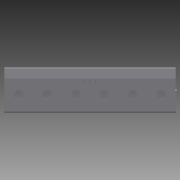
# Autodesk Inventor part: obodowka
Saved by Autodesk Inventor 2015 (Build 190159000, 159)
## iProperties
Created: 2015-09-19
Part Number: obodowka
Material: Generic
Document SubType Name: Sheet Metal
Designer: Komp
Density: 1 g/cm^3
Sheet Metal Rule: Default_mm
Appearance: Default
Flat Pattern Width: 17.082 cm
Flat Pattern Length: 30 cm
Flat Pattern Area: 512.46 cm^2
Sheet Metal Width: 170,820 mm
Sheet Metal Length: 300,000 mm
Sheet Metal Area: 51245,990 mm^2
Author: Komp
Autodesk Inventor part; units mm, degrees
ref_plane "YZ Plane" through (0, 0, 0) normal (1, 0, 0) x (0, 1, 0)
ref_plane "XZ Plane" through (0, 0, 0) normal (0, 1, 0) x (-1, 0, 0)
ref_plane "XY Plane" through (0, 0, 0) normal (0, 0, 1) x (1, 0, 0)
sketch "Sketch1" plane through (0, 0, 0) normal (1, 0, 0) x (0, 1, 0)
  line L0 (25, 40.1819) -> (25, 20.1819)
  line L1 (15, -39.8181) -> (-10, -39.8181)
  line L2 (-10, -39.8181) -> (-10, -19.8181)
  line L3 (25, 40.1819) -> (-10, 40.1819)
  line L4 (-10, 40.1819) -> (-10, 20.1819)
  line L5 (25, 20.1819) -> (15, -39.8181)
  point P0 (0, 0)
  dimension "d8" = 25
  dimension "d9" = 35
  dimension "d10" = 20
  dimension "d11" = 10
  dimension "d12" = 20
  dimension "d13" = 20
contour flange "Contour Flange1" sketch "Sketch1" thickness 1.5 bend radius 1.5 width 300 along (1, 0, 0) mid plane no both sides no wall seen from (0, -10, -29.8181) lies toward (0, 1, 0) curves L2 L1 L5 L0 L3 L4
bend "Bend1"
corner "Corner1"
sketch "Sketch3" plane through (0, -10, 20.1819) normal (0, -1, 0) x (1, 0, 0)
  line L0 (0, -57.4932) -> (0, -0.2449)
  line L1 (0, -58.5) -> (300, -58.5)
  line L2 (0, -40) -> (3, -40)
  line L3 (3, -40) -> (3, -58.5)
  line L4 (3, -58.5) -> (0, -58.5)
  line L5 (0, -58.5) -> (0, -40)
  point P0 (0, -20.1819)
  constraints: 8 end point, 2 parallel, 2 point on line, 1 horizontal, 1 perpendicular
extrude "Cut1" cut sketch "Sketch3" against normal blind 1.5
sketch "Sketch4" plane through (300, -10, -36.8181) normal (0, -1, 0) x (1, 0, 0)
  line L0 (0, 17) -> (-3, 17)
  line L1 (-3, 17) -> (-3, -1)
  line L2 (-3, -1) -> (0, -1)
  line L3 (0, -1) -> (0, 17)
  point P0 (-300, 36.8181)
  constraints: 8 end point, 2 parallel, 1 horizontal, 1 perpendicular
extrude "Cut2" cut sketch "Sketch4" against normal blind 1.5
sketch "Sketch5" plane through (0, -10, 20.1819) normal (0, -1, 0) x (1, 0, 0)
  line L0 (0, 0) -> (3, 0)
  line L1 (3, 0) -> (3, 19)
  line L2 (3, 19) -> (0, 19)
  line L3 (0, 19) -> (0, 0)
  point P0 (0, -20.1819)
  constraints: 8 end point, 2 parallel, 1 horizontal, 1 perpendicular
extrude "Cut3" cut sketch "Sketch5" against normal blind 1.5
sketch "Sketch6" plane through (300, -10, 20.1819) normal (0, -1, 0) x (1, 0, 0)
  line L0 (0, 0) -> (-3, 0)
  line L1 (-3, 0) -> (-3, 19)
  line L2 (-3, 19) -> (0, 19)
  line L3 (0, 19) -> (0, 0)
  point P0 (-300, -20.1819)
  constraints: 8 end point, 2 parallel, 1 horizontal, 1 perpendicular
extrude "Cut4" cut sketch "Sketch6" against normal blind 1.5
sketch "Sketch7" plane through (3, -10, 20.1819) normal (0, -1, 0) x (1, 0, 0)
  point P0 (-3, -20.1819)
hole "Hole1" at (20, -10, 28.1819) direction (0, 1, 0) diameter 2.5 depth 4.2 tip angle 118
hole "Hole2" at (20, -10, -27.8181) direction (0, 1, 0) diameter 2.5 depth 4.2 tip angle 118
hole "Hole3" at (280, -10, 28.1819) direction (0, 1, 0) diameter 2.5 depth 4.2 tip angle 118
hole "Hole4" at (280, -10, -27.8181) direction (0, 1, 0) diameter 2.5 depth 4.2 tip angle 118
hole "Hole5" at (150, -10, 28.1819) direction (0, 1, 0) diameter 2.5 depth 4.2 tip angle 118
hole "Hole6" at (150, -10, -27.8181) direction (0, 1, 0) diameter 2.5 depth 4.2 tip angle 118
hole "Hole7" at (275, 20.3498, -7.7195) direction (0, -0.9863939, 0.164399) diameter 16 depth 1.5 tip angle 118
hole "Hole8" at (225, 20.3498, -7.7195) direction (0, -0.9863939, 0.164399) diameter 16 depth 1.5 tip angle 118
hole "Hole9" at (175, 20.3498, -7.7195) direction (0, -0.9863939, 0.164399) diameter 16 depth 1.5 tip angle 118
hole "Hole10" at (25, 20.3498, -7.7195) direction (0, -0.9863939, 0.164399) diameter 16 depth 1.5 tip angle 118
hole "Hole11" at (75, 20.3498, -7.7195) direction (0, -0.9863939, 0.164399) diameter 16 depth 1.5 tip angle 118
hole "Hole12" at (275, 25, 30.1819) direction (0, -1, 0) diameter 3 depth 1.5 tip angle 118
hole "Hole13" at (225, 25, 30.1819) direction (0, -1, 0) diameter 3 depth 1.5 tip angle 118
hole "Hole14" at (175, 25, 30.1819) direction (0, -1, 0) diameter 3 depth 1.5 tip angle 118
hole "Hole15" at (75, 25, 30.1819) direction (0, -1, 0) diameter 3 depth 1.5 tip angle 118
hole "Hole16" at (25, 25, 30.1819) direction (0, -1, 0) diameter 3 depth 1.5 tip angle 118
hole "Hole18" at (160, 24.1372, 15.005) direction (0, -0.9863939, 0.164399) diameter 3 depth 1.5 tip angle 118
hole "Hole19" at (150, 24.1372, 15.005) direction (0, -0.9863939, 0.164399) diameter 3 depth 1.5 tip angle 118
hole "Hole20" at (140, 24.1372, 15.005) direction (0, -0.9863939, 0.164399) diameter 3 depth 1.5 tip angle 118
hole "Hole22" at (125, 20.3498, -7.7195) direction (0, -0.9863939, 0.164399) diameter 16 depth 1.5 tip angle 118
hole "Hole23" at (125, 25, 29.937) direction (0, -1, 0) diameter 3 depth 1.5 tip angle 118
sketch "Sketch2" plane through (297, 150.427, -1.5) normal (0, 0, -1) x (-1, 0, 0)
  line L0 (297, -17) -> (294, -17)
  line L1 (294, -17) -> (294, -18.131)
  line L2 (294, -18.131) -> (297, -18.131)
  line L3 (297, -18.131) -> (297, -17)
  constraints: 8 end point, 2 parallel, 1 horizontal, 1 perpendicular
equation "\"d24\" = Thickness"
equation "\"d26\" = Thickness"
equation "\"d28\" = Thickness"
equation "\"d30\" = Thickness"
equation "\"d93\" = Thickness"
equation "\"d102\" = Thickness"
equation "\"d111\" = Thickness"
equation "\"d120\" = Thickness"
equation "\"d129\" = Thickness"
equation "\"d138\" = Thickness"
equation "\"d147\" = Thickness"
equation "\"d156\" = Thickness"
equation "\"d165\" = Thickness"
equation "\"d174\" = Thickness"
equation "\"d197\" = Thickness"
equation "\"d206\" = Thickness"
equation "\"d215\" = Thickness"
equation "\"d233\" = Thickness"
equation "\"d14\" = BendReliefWidth"
equation "\"d15\" = BendReliefDepth"
equation "\"d16\" = MinimumRemnant"
equation "\"d17\" = BendRadius"
equation "\"d19\" = BendRadius"
equation "\"d21\" = CornerReliefSize"
equation "\"d22\" = GapSize"
equation "\"d23\" = JacobiRadiusSize"
equation "\"BendRadius\" = Thickness"
equation "\"BendReliefWidth\" = Thickness"
equation "\"BendReliefDepth\" = 0.5 * Thickness"
equation "\"CornerReliefSize\" = 4 * Thickness"
equation "\"MinimumRemnant\" = 2 * Thickness"
equation "\"TransitionRadius\" = BendRadius"
equation "\"JacobiRadiusSize\" = BendRadius"
equation "\"GapSize\" = Thickness"
equation "\"d0\" = Thickness"
equation "\"d2\" = Thickness"
equation "\"d4\" = Thickness"
equation "\"d6\" = Thickness"
equation "\"Thickness\" = 1.5"
body "Solid1"
